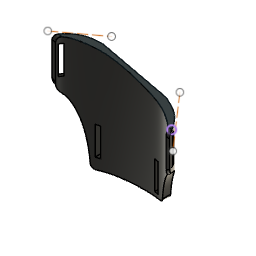
Back Hand Exo v4 v4 (Autodesk Fusion 360 design; units mm, degrees)
Autodesk Fusion 360 part; units mm, degrees
sketch "Base" plane through (0, 0, 0) normal (0, 0, 1) x (1, 0, 0)
  spline S0 degree 5 poles (13.752, -0.0001) (13.9653, 0.7958) (14.5381, 2.2842) (15.837, 4.206) (18.3493, 6.2617) (22.4599, 8.449) (27.2985, 10.6406) (33.3248, 12.6283) (41.3156, 13.6872) (50.5233, 13.835) (59.8574, 13.2455) (67.9918, 12.2717) (74.1601, 11.1616) (78.0856, 10.0513) (81.6903, 8.4944) (86.1249, 6.1568) (89.3627, 3.8311) (90.983, 1.9475) (91.5765, 0.6553) (91.752, 0) knots 0 0 0 0 0 0 0.066667 0.133333 0.2 0.266667 0.333333 0.4 0.466667 0.533333 0.6 0.666667 0.733333 0.8 0.866667 0.933333 1 1 1 1 1 1
  line L0 (11.7287, -7.5513) -> (15.7754, 7.551)
  line L1 (0, 0) -> (130, 0) construction
  line L2 (90.0188, 6.4684) -> (93.4853, -6.4684)
  line L3 (72.0197, 12) -> (83.6365, 8)
  line L4 (20.3175, 8.0956) -> (37.1866, 13.9041)
  line L5 (28.752, 32.4834) -> (28.752, -47.2676) construction
  line L6 (79.3904, 33.3073) -> (79.3904, -47.7619) construction
  line L7 (13.752, -0.0001) -> (11.252, 0)
  line L8 (94.252, 0) -> (91.752, 0)
  line L9 (30.252, 16.6538) -> (75.252, 16.6538)
  line L10 (52.752, 16.6538) -> (52.752, -22.3142) construction
  spline S1 degree 5 poles (11.252, 0) (11.5338, 0.5886) (12.1054, 1.7418) (12.9869, 3.3999) (14.2112, 5.465) (15.8292, 7.788) (17.544, 9.832) (19.3661, 11.5801) (21.3048, 13.0286) (23.3626, 14.2079) (25.537, 15.1728) (27.3674, 15.819) (28.7903, 16.2536) (29.7611, 16.5237) (30.252, 16.6538) knots 0 0 0 0 0 0 0.1 0.2 0.3 0.4 0.5 0.6 0.7 0.8 0.9 1 1 1 1 1 1
  spline S2 degree 5 poles (75.252, 16.6538) (75.631, 16.4987) (76.3973, 16.1962) (77.5715, 15.7657) (79.1807, 15.218) (81.2306, 14.4657) (83.2776, 13.5113) (85.2833, 12.2312) (87.2246, 10.5613) (89.093, 8.4929) (90.8878, 6.0413) (92.267, 3.7932) (93.2711, 1.9548) (93.9273, 0.6627) (94.252, 0) knots 0 0 0 0 0 0 0.1 0.2 0.3 0.4 0.5 0.6 0.7 0.8 0.9 1 1 1 1 1 1
  line L11 (26.8617, 15.7552) -> (33.6424, 17.5524)
  line L12 (72.1212, 17.9353) -> (78.3829, 15.3723)
  point P0 (28.752, 10.9999)
  point P1 (77.8281, 10)
  point P2 (20, 12)
  point P3 (84, 13)
  dimension "d1" = 78
  dimension "d3" = 15
  dimension "d4" = 11
  dimension "d5" = 10
  dimension "d6" = 75
  dimension "d7" = 75
  dimension "d8" = 19
  dimension "d9" = 19
  dimension "d10" = 2.5
  dimension "d11" = 2.5
  dimension "d71" = 45
  dimension "d72" = 39
  constraint midpoint S0.start L0
  constraint coincident L1.start origin
  constraint horizontal L1
  constraint midpoint S0.end L2
  constraint midpoint P1 L3
  constraint midpoint P0 L4
  constraint coincident L1 L7.end
  constraint coincident L1 L8.start
  constraint perpendicular L1 L5
  constraint vertical L6
  constraint coincident P0 L5
  constraint coincident S0.end L1
  constraint perpendicular L5 L9
  constraint vertical L10
  constraint midpoint L9 L10.start
  constraint midpoint L9.start L11
  constraint midpoint L9.end L12
  measures "d1" distance of S0.start S0.end
  measures "d3" distance of S0.start P0
  measures "d4" distance of S0.start P0
  measures "d5" distance of P1 S0.end
  measures "d6" angle of L0 L1
  measures "d7" angle of L1 L2
  measures "d8" angle of L1 L3
  measures "d9" angle of L1 L4
  measures "d10" distance of S0.end L8.start
  measures "d11" distance of S0.start L7.end
  measures "d71" distance of L9.start L9.end
  measures "d72" distance of S0.start L10
extrude "Extrude1" add sketch "Base" along normal blind 80
ref_plane "WorkPlane1" through (0, 34, 0) normal (0, 1, 0) x (0, 0, 1)
ref_plane "WorkPlane2" through (0, -2, 0) normal (0, 1, 0) x (0, 0, 1)
sketch "Bottom cut" plane through (0, -2, 0) normal (0, 1, 0) x (1, 0, 0)
  line L0 (104.8084, -94.0595) -> (104.8084, 16.0436) construction
  line L1 (124.2592, 0) -> (-25.481, 0) construction
  line L2 (7.8084, -95.0569) -> (7.8084, 27.3148) construction
  line L3 (10.7244, 0) -> (10.7244, -80) construction
  line L4 (100.7244, 0) -> (100.7244, -80) construction
  line L5 (-40, -55.0042) -> (-40, 40)
  line L6 (-40, 40) -> (120, 40)
  line L7 (120, 40) -> (120, -40)
  line L8 (120, -40) -> (104.8084, -39.0079)
  spline S0 degree 5 poles (4.5707, -55.0042) (5.4547, -54.2774) (7.185, -52.7903) (9.6672, -50.4587) (12.7463, -47.1447) (16.1864, -42.6382) (19.185, -37.7387) (21.7128, -32.42) (23.7655, -26.6781) (25.3732, -20.5401) (26.5747, -14.0405) (27.2401, -8.5774) (27.5837, -4.3416) (27.7449, -1.4573) (27.8084, 0) knots 0 0 0 0 0 0 0.1 0.2 0.3 0.4 0.5 0.6 0.7 0.8 0.9 1 1 1 1 1 1
  spline S1 degree 5 poles (104.8084, -39.0079) (103.8636, -38.7543) (102.0133, -38.2112) (99.3558, -37.2887) (96.0521, -35.8397) (92.3487, -33.6388) (89.108, -31.015) (86.3653, -27.9361) (84.1353, -24.3885) (82.3927, -20.3954) (81.0985, -15.9925) (80.3914, -12.1701) (80.0338, -9.1455) (79.871, -7.06) (79.8084, -6) knots 0 0 0 0 0 0 0.1 0.2 0.3 0.4 0.5 0.6 0.7 0.8 0.9 1 1 1 1 1 1
  line L9 (79.8084, -6) -> (27.8084, 0)
  line L10 (4.5707, -55.0042) -> (-40, -55.0042)
  point P0 (20.8084, -34.1255)
  point P1 (86.8084, -28.2303)
  dimension "d50" = 20
  dimension "d51" = 13
  dimension "d52" = 18
  dimension "d53" = 25
  dimension "d54" = 97
  dimension "d55" = 6
  constraint vertical L0
  constraint perpendicular L0 L1
  constraint perpendicular L1 L2
  constraint coincident origin L1
  constraint coincident L0 L8.end
  constraint perpendicular L5 L6
  constraint perpendicular L6 L7
  constraint vertical L5
  constraint perpendicular L5 L10
  constraint coincident L1 S0.end
  constraint midpoint L0 L8.end
  measures "d50" distance of L2 S0.end
  measures "d51" distance of L2 P0
  measures "d52" distance of L0 P1
  measures "d53" distance of L0 S1.end
  measures "d54" distance of L0 L2
  measures "d55" distance of L1 S1.end
sketch "Top cut" plane through (0, -2, 0) normal (0, 1, 0) x (1, 0, 0)
  line L0 (101.7244, -58) -> (2.8084, -81)
  line L1 (2.8084, -81) -> (2.8084, -105)
  line L2 (2.8084, -105) -> (101.7244, -105)
  line L3 (101.7244, -105) -> (101.7244, -58)
  line L4 (100.7244, -80) -> (10.7244, -80)
  line L5 (7.8084, -95.0569) -> (7.8084, 27.3148)
  line L6 (100.7244, 0) -> (100.7244, -80)
  dimension "d41" = 22
  dimension "d42" = 1
  dimension "d43" = 5
  dimension "d44" = 25
  dimension "d49" = 1
  constraint vertical L1
  constraint perpendicular L1 L2
  constraint perpendicular L2 L3
  measures "d41" distance of L0.start L4
  measures "d42" distance of L0.end L4
  measures "d43" distance of L1 L5
  measures "d44" distance of L2 L4
  measures "d49" distance of L3 L6
extrude "Extrude4" cut sketch "Bottom cut" along normal blind 40
extrude "Extrude5" cut sketch "Top cut" along normal blind 55
fillet "Fillet5" radius 3 6 edges at (27.8084, 13.3008, 0) (79.8084, 12.1091, 6) (12.502, -0.0001, 78.746) (93.002, 0, 60.0281) (12.5265, -0.0001, 47.1929) (92.9812, 0, 33.8848)
sketch "Strap holes1-2" plane through (0, 16.6538, 0) normal (0, 1, 0) x (-1, 0, 0)
  spline S0 degree 3 poles (-30.252, 0.3696) (-30.2872, 0.3651) (-30.3224, 0.3613) (-30.5631, 0.3393) (-30.7699, 0.3417) (-30.9749, 0.3654) knots 0.051258 0.051258 0.051258 0.051258 0.061889 0.061889 0.123778 0.123778 0.123778 0.123778
  line L0 (-30.252, 0.3696) -> (-30.252, 74.6188)
  line L1 (-30.252, 74.6188) -> (-75.252, 64.1554)
  line L2 (-75.252, 64.1554) -> (-75.252, 5.4743)
  line L3 (-75.252, 5.4743) -> (-30.9749, 0.3654)
  line L4 (-75.252, 28) -> (-72.252, 28)
  line L5 (-72.252, 28) -> (-72.252, 8)
  line L6 (-72.252, 8) -> (-75.252, 8)
  line L7 (-75.252, 8) -> (-75.252, 28)
  line L8 (-33.252, 28) -> (-30.252, 28)
  line L9 (-30.252, 28) -> (-30.252, 8)
  line L10 (-30.252, 8) -> (-33.252, 8)
  line L11 (-33.252, 8) -> (-33.252, 28)
  dimension "d86" = 20
  dimension "d87" = 8
  dimension "d88" = 8
  dimension "d89" = 3
  constraint horizontal L4
  constraint vertical L5
  constraint horizontal L6
  constraint vertical L7
  constraint horizontal L8
  constraint vertical L9
  constraint horizontal L10
  constraint vertical L11
  constraint equal L5 L9
  constraint equal L6 L10
  constraint collinear L2 L7
  constraint collinear L0 L9
  measures "d86" distance of L8.end L9.end
  measures "d87" distance of origin L6
  measures "d88" distance of origin L10
  measures "d89" distance of L8.start L8.end
extrude "Extrude9" cut sketch "Strap holes1-2" against normal blind 12 contours L0 L8 L9 L10 L11 | L2 L4 L5 L6 L7
sketch "Construction lines" plane through (18.0122, 0, 77.4648) normal (0.226479, 0, 0.974016) x (0, 1, 0)
  line L0 (3, -73.8013) -> (3, -76.6575)
  spline S0 degree 3 poles (16.6538, -58.7669) (15.8139, -60.8738) (15.3084, -62.6333) (13.7959, -66.4997) (12.7514, -68.5403) (8.7557, -72.9177) (6.0876, -74.8715) (3, -76.6575) knots -3.463321 -3.463321 -3.463321 -3.463321 -2.542901 -2.542901 -1.469021 -1.469021 -0.348561 -0.348561 -0.348561 -0.348561
  line L1 (16.6538, -58.7669) -> (16.6538, -12.5664)
  spline S1 degree 3 poles (3, 5.3518) (4.4398, 4.5288) (5.8451, 3.6285) (9.4992, 0.8936) (11.0843, -0.7862) (13.6108, -4.229) (15.2503, -7.1298) (16.6538, -12.5664) knots -3.904923 -3.904923 -3.904923 -3.904923 -3.114185 -3.114185 -1.684445 -1.684445 0 0 0 0
  line L2 (3, 5.3518) -> (2.9998, 2.9242)
  spline S2 degree 3 poles (3, -73.8013) (3.7027, -73.1055) (4.3459, -72.2992) (6.4441, -69.3508) (7.7722, -66.7548) (9.2291, -63.5462) (9.772, -62.1746) (12.4028, -53.6965) (13.5824, -40.3684) (13.809, -19.6639) (12.0211, -13.2463) (9.1223, -6.1584) (7.6302, -2.7127) (5.085, 0.9851) (4.2261, 1.9685) (3.156, 2.8074) (3.0782, 2.8665) (2.9998, 2.9242) knots -6.903103 -6.903103 -6.903103 -6.903103 -6.723866 -6.723866 -6.232481 -6.232481 -5.876872 -5.876872 -4.173273 -4.173273 -1.579181 -1.579181 -0.749477 -0.749477 -0.371417 -0.371417 -0.342017 -0.342017 -0.342017 -0.342017
  line L3 (0, 10) -> (24.0161, -11.5563) construction
  line L4 (25, -60) -> (-7.1736, -87.8504) construction
ref_plane "WorkPlane3" through (18.7701, 12.0081, 77.2886) normal (0.752855, -0.658187, 0) x (0.650612, 0.74419, -0.151281)
ref_plane "WorkPlane4" through (90.0165, 8.9132, 60.7223) normal (-0.764523, -0.644597, 0) x (0.637476, -0.756077, -0.148226)
sketch "Strap hole3" plane through (18.7701, 12.0081, 77.2886) normal (0.752855, -0.658187, 0) x (0.650612, 0.74419, -0.151281)
  line L0 (-16.1358, 0) -> (16.1358, 0)
  line L1 (-14.3189, 1.0938) -> (-8.2677, -38.4458) construction
  line L2 (-10.1527, -26.1289) -> (-13.6261, -3.4328) construction
  line L3 (-10.3799, -4.8256) -> (-7.3543, -24.5954)
  line L4 (-7.3543, -24.5954) -> (-4.3889, -24.1416)
  line L5 (-4.3889, -24.1416) -> (-7.4145, -4.3718)
  line L6 (-7.4145, -4.3718) -> (-10.3799, -4.8256)
  dimension "d97" = 40
  dimension "d98" = 20
  dimension "d99" = 3
  constraint parallel L1 L2
  constraint collinear L1 L2
  constraint parallel L1 L3
  constraint perpendicular L3 L4
  constraint perpendicular L3 L6
  constraint parallel L3 L5
  measures "d97" distance of L1.start L1.end
  measures "d98" distance of L3.start L3.end
  measures "d99" distance of L3.end L4.end
extrude "Extrude10" cut sketch "Strap hole3" along normal blind 15
sketch "Strap hole4" plane through (90.0165, 8.9132, 60.7223) normal (-0.764523, -0.644597, 0) x (0.637476, -0.756077, -0.148226)
  line L0 (8.5937, 7.0554) -> (14.6402, -33.2862) construction
  line L1 (12.7879, -20.9277) -> (10.0417, -2.6052) construction
  line L2 (6.0688, -3.0847) -> (9.0334, -22.8638)
  line L3 (6.0688, -3.0847) -> (3.102, -3.5294)
  line L4 (3.102, -3.5294) -> (6.0665, -23.3084)
  line L5 (6.0665, -23.3084) -> (9.0334, -22.8638)
  dimension "d102" = 20
  dimension "d103" = 4
  dimension "d104" = 4
  dimension "d105" = 3
  constraint collinear L0 L1
  constraint perpendicular L2 L3
  constraint perpendicular L3 L4
  constraint perpendicular L4 L5
  measures "d102" distance of L2.start L2.end
  measures "d103" distance of L0 L2.end
  measures "d104" distance of L0 L2.start
  measures "d105" distance of L2.start L3.end
extrude "Extrude11" cut sketch "Strap hole4" along normal blind 20
equation "d72 = ( 78 / 2 ) * 1 mm"
